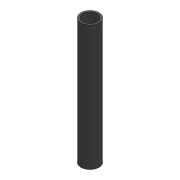
# Autodesk Inventor part: 11_019_TIBIA_CFRP_PIPE_R1
Saved by Autodesk Inventor 2021.2 (Build 252289000, 289)
## iProperties
Created: 2018-02-01
Part Number: 11_019_TIBIA_CFRP_PIPE_R1
Material: CFRP
Document SubType Name: Modeling
Designer: y6tada
Density: 1.43 g/cm^3
Appearance: カーボンファイバー
Mass: 2.81207 g
Surface Area: 39.8951 cm^2
Volume: 1.96648 cm^3
Author: y6tada
Autodesk Inventor part; units mm, degrees
ref_plane "YZ Plane" through (0, 0, 0) normal (1, 0, 0) x (0, 1, 0)
ref_plane "XZ Plane" through (0, 0, 0) normal (0, 1, 0) x (-1, 0, 0)
ref_plane "XY Plane" through (0, 0, 0) normal (0, 0, 1) x (1, 0, 0)
sketch "スケッチ2" plane through (0, 0, 0) normal (0, 0, 1) x (1, 0, 0)
  circle A0 centre (0, 0) radius 4
  circle A1 centre (0, 0) radius 5
  dimension "d3" = 8
  dimension "d4" = 10
  constraints: 2 centre point, 2 coincident
  measures "d3" diameter of A0
  measures "d4" diameter of A1
extrude "押し出し1" add sketch "スケッチ2" against normal blind 69.55
